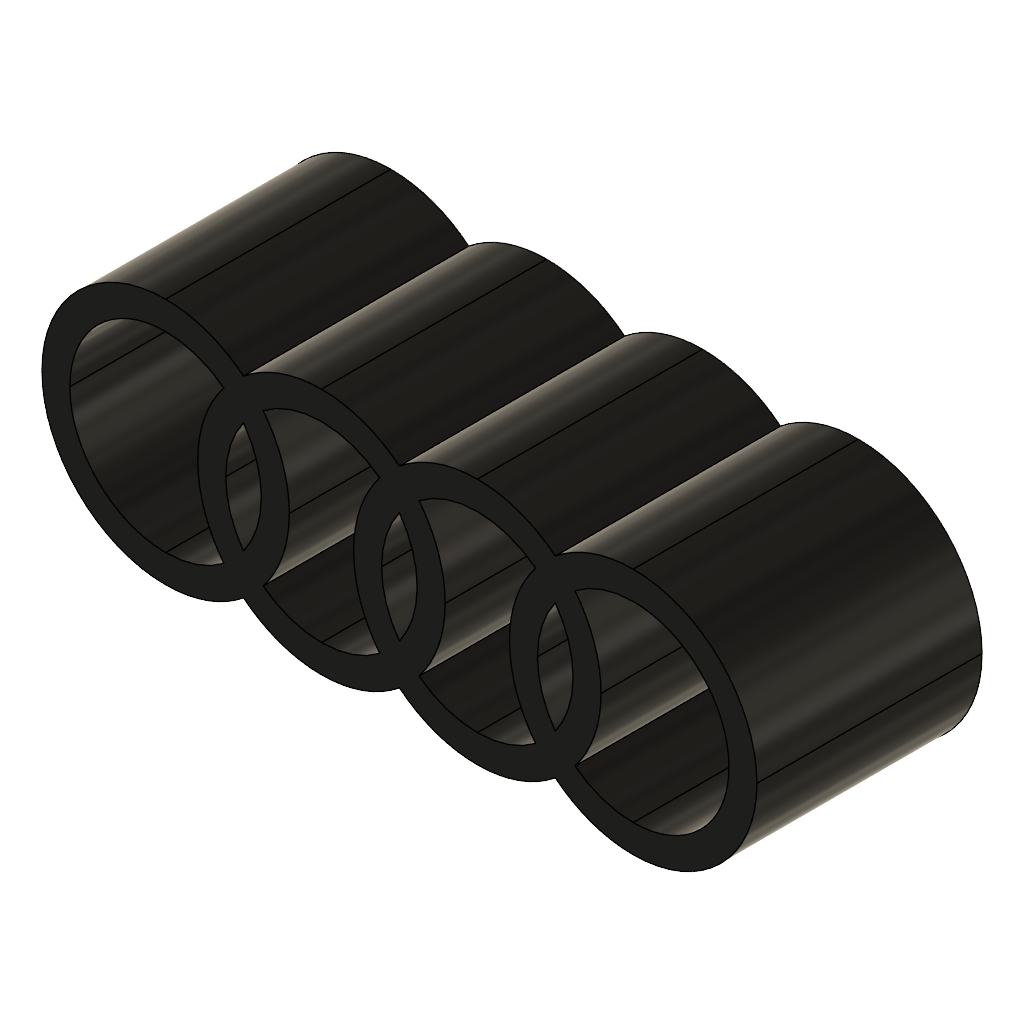
AudiLogo (Autodesk Fusion 360 design; units mm, degrees)
part number: 2026-10-03-23-30-38-070
Autodesk Fusion 360 part; units mm, degrees
sketch "Sketch1" plane through (0, 0, 0) normal (0, 1, 0) x (1, 0, 0)
  spline S0 degree 3 poles (2.0714, 1.1235) (1.809, 1.1235) (1.5682, 1.0315) (1.3793, 0.878) knots 0 0 0 0 1 1 1 1
  spline S1 degree 3 poles (1.3793, 0.878) (1.1904, 1.0315) (0.9496, 1.1235) (0.6872, 1.1235) knots 0 0 0 0 1 1 1 1
  spline S2 degree 3 poles (0.6872, 1.1235) (0.4247, 1.1235) (0.1839, 1.0315) (-0.005, 0.878) knots 0 0 0 0 1 1 1 1
  spline S3 degree 3 poles (-0.005, 0.878) (-0.1939, 1.0315) (-0.4347, 1.1235) (-0.6972, 1.1235) knots 0 0 0 0 1 1 1 1
  spline S4 degree 3 poles (-0.6972, 1.1235) (-0.9596, 1.1235) (-1.2004, 1.0315) (-1.3893, 0.878) knots 0 0 0 0 1 1 1 1
  spline S5 degree 3 poles (-1.3893, 0.878) (-1.5782, 1.0315) (-1.819, 1.1235) (-2.0815, 1.1235) knots 0 0 0 0 1 1 1 1
  spline S6 degree 3 poles (-2.0815, 1.1235) (-2.6881, 1.1235) (-3.18, 0.6317) (-3.18, 0.025) knots 0 0 0 0 1 1 1 1
  spline S7 degree 3 poles (-3.18, 0.025) (-3.18, -0.5817) (-2.6881, -1.0736) (-2.0815, -1.0736) knots 0 0 0 0 1 1 1 1
  spline S8 degree 3 poles (-2.0815, -1.0736) (-1.819, -1.0736) (-1.5782, -0.9815) (-1.3893, -0.828) knots 0 0 0 0 1 1 1 1
  spline S9 degree 3 poles (-1.3893, -0.828) (-1.2004, -0.9815) (-0.9596, -1.0736) (-0.6972, -1.0736) knots 0 0 0 0 1 1 1 1
  spline S10 degree 3 poles (-0.6972, -1.0736) (-0.4347, -1.0736) (-0.1939, -0.9815) (-0.005, -0.828) knots 0 0 0 0 1 1 1 1
  spline S11 degree 3 poles (-0.005, -0.828) (0.1839, -0.9815) (0.4247, -1.0736) (0.6872, -1.0736) knots 0 0 0 0 1 1 1 1
  spline S12 degree 3 poles (0.6872, -1.0736) (0.9496, -1.0736) (1.1904, -0.9815) (1.3793, -0.828) knots 0 0 0 0 1 1 1 1
  spline S13 degree 3 poles (1.3793, -0.828) (1.5682, -0.9815) (1.809, -1.0736) (2.0714, -1.0736) knots 0 0 0 0 1 1 1 1
  spline S14 degree 3 poles (2.0714, -1.0736) (2.6781, -1.0736) (3.17, -0.5817) (3.17, 0.025) knots 0 0 0 0 1 1 1 1
  spline S15 degree 3 poles (3.17, 0.025) (3.17, 0.6317) (2.6781, 1.1235) (2.0714, 1.1235) knots 0 0 0 0 1 1 1 1
  spline S16 degree 3 poles (1.3793, -0.4687) (1.2798, -0.3295) (1.2211, -0.1592) (1.2211, 0.025) knots 0 0 0 0 1 1 1 1
  spline S17 degree 3 poles (1.2211, 0.025) (1.2211, 0.2092) (1.2798, 0.3795) (1.3793, 0.5187) knots 0 0 0 0 1 1 1 1
  spline S18 degree 3 poles (1.3793, 0.5187) (1.4788, 0.3795) (1.5375, 0.2092) (1.5375, 0.025) knots 0 0 0 0 1 1 1 1
  spline S19 degree 3 poles (1.5375, 0.025) (1.5375, -0.1592) (1.4788, -0.3295) (1.3793, -0.4687) knots 0 0 0 0 1 1 1 1
  spline S20 degree 3 poles (-0.005, -0.4687) (-0.1045, -0.3295) (-0.1632, -0.1592) (-0.1632, 0.025) knots 0 0 0 0 1 1 1 1
  spline S21 degree 3 poles (-0.1632, 0.025) (-0.1632, 0.2092) (-0.1045, 0.3795) (-0.005, 0.5187) knots 0 0 0 0 1 1 1 1
  spline S22 degree 3 poles (-0.005, 0.5187) (0.0945, 0.3795) (0.1532, 0.2092) (0.1532, 0.025) knots 0 0 0 0 1 1 1 1
  spline S23 degree 3 poles (0.1532, 0.025) (0.1532, -0.1592) (0.0945, -0.3295) (-0.005, -0.4687) knots 0 0 0 0 1 1 1 1
  spline S24 degree 3 poles (-1.3893, -0.4687) (-1.4888, -0.3295) (-1.5475, -0.1592) (-1.5475, 0.025) knots 0 0 0 0 1 1 1 1
  spline S25 degree 3 poles (-1.5475, 0.025) (-1.5475, 0.2092) (-1.4888, 0.3795) (-1.3893, 0.5187) knots 0 0 0 0 1 1 1 1
  spline S26 degree 3 poles (-1.3893, 0.5187) (-1.2898, 0.3795) (-1.2311, 0.2092) (-1.2311, 0.025) knots 0 0 0 0 1 1 1 1
  spline S27 degree 3 poles (-1.2311, 0.025) (-1.2311, -0.1592) (-1.2898, -0.3295) (-1.3893, -0.4687) knots 0 0 0 0 1 1 1 1
  spline S28 degree 3 poles (-2.9318, 0.025) (-2.9318, 0.4946) (-2.5511, 0.8754) (-2.0815, 0.8754) knots 0 0 0 0 1 1 1 1
  spline S29 degree 3 poles (-2.0815, 0.8754) (-1.8867, 0.8754) (-1.7073, 0.8098) (-1.5639, 0.6994) knots 0 0 0 0 1 1 1 1
  spline S30 degree 3 poles (-1.5639, 0.6994) (-1.7089, 0.5134) (-1.7957, 0.2793) (-1.7957, 0.025) knots 0 0 0 0 1 1 1 1
  spline S31 degree 3 poles (-1.7957, 0.025) (-1.7957, -0.2293) (-1.7089, -0.4634) (-1.5639, -0.6494) knots 0 0 0 0 1 1 1 1
  spline S32 degree 3 poles (-1.5639, -0.6494) (-1.7073, -0.7595) (-1.8867, -0.8254) (-2.0815, -0.8254) knots 0 0 0 0 1 1 1 1
  spline S33 degree 3 poles (-2.0815, -0.8254) (-2.5511, -0.8254) (-2.9318, -0.4446) (-2.9318, 0.025) knots 0 0 0 0 1 1 1 1
  spline S34 degree 3 poles (-1.2147, -0.6494) (-1.0697, -0.4634) (-0.9829, -0.2293) (-0.9829, 0.025) knots 0 0 0 0 1 1 1 1
  spline S35 degree 3 poles (-0.9829, 0.025) (-0.9829, 0.2793) (-1.0697, 0.5134) (-1.2147, 0.6994) knots 0 0 0 0 1 1 1 1
  spline S36 degree 3 poles (-1.2147, 0.6994) (-1.0713, 0.8095) (-0.8919, 0.8754) (-0.6972, 0.8754) knots 0 0 0 0 1 1 1 1
  spline S37 degree 3 poles (-0.6972, 0.8754) (-0.5024, 0.8754) (-0.323, 0.8098) (-0.1796, 0.6994) knots 0 0 0 0 1 1 1 1
  spline S38 degree 3 poles (-0.1796, 0.6994) (-0.3249, 0.5132) (-0.4114, 0.2793) (-0.4114, 0.025) knots 0 0 0 0 1 1 1 1
  spline S39 degree 3 poles (-0.4114, 0.025) (-0.4114, -0.2293) (-0.3246, -0.4634) (-0.1796, -0.6494) knots 0 0 0 0 1 1 1 1
  spline S40 degree 3 poles (-0.1796, -0.6494) (-0.323, -0.7595) (-0.5024, -0.8254) (-0.6972, -0.8254) knots 0 0 0 0 1 1 1 1
  spline S41 degree 3 poles (-0.6972, -0.8254) (-0.8919, -0.8254) (-1.0713, -0.7598) (-1.2147, -0.6494) knots 0 0 0 0 1 1 1 1
  spline S42 degree 3 poles (0.1696, -0.6494) (0.3149, -0.4632) (0.4014, -0.2293) (0.4014, 0.025) knots 0 0 0 0 1 1 1 1
  spline S43 degree 3 poles (0.4014, 0.025) (0.4014, 0.2793) (0.3146, 0.5134) (0.1696, 0.6997) knots 0 0 0 0 1 1 1 1
  spline S44 degree 3 poles (0.1696, 0.6997) (0.313, 0.8098) (0.4924, 0.8756) (0.6872, 0.8756) knots 0 0 0 0 1 1 1 1
  spline S45 degree 3 poles (0.6872, 0.8756) (0.8819, 0.8756) (1.0613, 0.81) (1.2047, 0.6997) knots 0 0 0 0 1 1 1 1
  spline S46 degree 3 poles (1.2047, 0.6997) (1.0594, 0.5134) (0.9729, 0.2795) (0.9729, 0.0253) knots 0 0 0 0 1 1 1 1
  spline S47 degree 3 poles (0.9729, 0.0253) (0.9729, -0.229) (1.0597, -0.4632) (1.2047, -0.6492) knots 0 0 0 0 1 1 1 1
  spline S48 degree 3 poles (1.2047, -0.6492) (1.0613, -0.7592) (0.8819, -0.8251) (0.6872, -0.8251) knots 0 0 0 0 1 1 1 1
  spline S49 degree 3 poles (0.6872, -0.8251) (0.4924, -0.8254) (0.313, -0.7598) (0.1696, -0.6494) knots 0 0 0 0 1 1 1 1
  spline S50 degree 3 poles (2.0714, -0.8254) (1.8767, -0.8254) (1.6973, -0.7598) (1.5539, -0.6494) knots 0 0 0 0 1 1 1 1
  spline S51 degree 3 poles (1.5539, -0.6494) (1.6989, -0.4632) (1.7857, -0.2293) (1.7857, 0.025) knots 0 0 0 0 1 1 1 1
  spline S52 degree 3 poles (1.7857, 0.025) (1.7857, 0.2793) (1.6989, 0.5134) (1.5539, 0.6994) knots 0 0 0 0 1 1 1 1
  spline S53 degree 3 poles (1.5539, 0.6994) (1.6973, 0.8095) (1.8767, 0.8754) (2.0714, 0.8754) knots 0 0 0 0 1 1 1 1
  spline S54 degree 3 poles (2.0714, 0.8754) (2.5411, 0.8754) (2.9218, 0.4946) (2.9218, 0.025) knots 0 0 0 0 1 1 1 1
  spline S55 degree 3 poles (2.9218, 0.025) (2.9218, -0.4446) (2.5411, -0.8254) (2.0714, -0.8254) knots 0 0 0 0 1 1 1 1
extrude "Extrude1" add sketch "Sketch1" along normal blind 2
